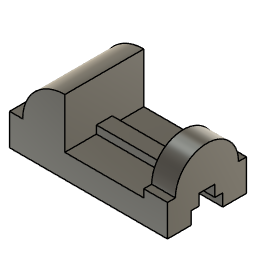
task 1 object 2 (Autodesk Fusion 360 design; units mm, degrees)
Autodesk Fusion 360 part; units mm, degrees
sketch "Sketch1" plane through (0, 0, 0) normal (0, 0, 1) x (1, 0, 0)
  line L0 (0, 0) -> (200, 0)
  line L1 (200, 0) -> (200, -100)
  line L2 (200, -100) -> (0, -100)
  line L3 (0, -100) -> (0, 0)
  dimension "d1" = 200
  dimension "d2" = 100
  constraint horizontal L0
  constraint vertical L1
  constraint horizontal L2
  constraint vertical L3
  constraint coincident L0.start L3.end
  measures "d1" distance of L0.start L0.end
  measures "d2" distance of L0.start L2.end
extrude "Extrude1" add sketch "Sketch1" along normal blind 40
sketch "Sketch2" plane through (0, 0, 40) normal (0, 0, 1) x (-1, 0, 0)
  line L0 (0, 100) -> (-200, 100)
  line L1 (-200, 100) -> (-200, 0)
  line L2 (-200, 0) -> (0, 0)
  line L3 (0, 0) -> (0, 100)
  line L4 (-200, 0) -> (-170, 0)
  line L5 (-170, 100) -> (-170, 0)
  line L6 (-200, 100) -> (-170, 100)
  constraint coincident L1.end L2.start
  constraint coincident L2 L4.end
  constraint coincident L0 L5.start
  constraint perpendicular L4 L5
  constraint coincident L0.end L1.start
extrude "Extrude2" add sketch "Sketch2" along normal blind 40 contours L0 L1 L2 L4 L5 L6
sketch "Sketch3" plane through (170, 0, 0) normal (-1, 0, 0) x (0, -1, 0)
  line L0 (0, 40) -> (100, 40)
  line L1 (100, 40) -> (100, 80)
  line L2 (100, 80) -> (0, 80)
  line L3 (0, 80) -> (0, 40)
  arc A0 (90, 40) -> (10, 40) centre (50, 40) ccw
  dimension "d7" = 80
  constraint midpoint L0 A0.centre
  constraint coincident L0 A0.end
  constraint coincident L0 A0.start
  measures "d7" diameter of A0
extrude "Extrude3" cut sketch "Sketch3" against normal blind 30 contours L0 L2 L3 A0 | L0 L1 L2 A0
sketch "Sketch4" plane through (0, 0, 0) normal (-1, 0, 0) x (0, -1, 0)
  line L0 (0, 0) -> (100, 0)
  line L1 (100, 0) -> (100, 40)
  line L2 (100, 40) -> (0, 40)
  line L3 (0, 40) -> (0, 0)
  line L4 (50, 30) -> (40, 30)
  line L5 (40, 30) -> (40, 15.5434)
  line L6 (40, 15.5434) -> (30, 15.5434)
  line L7 (30, 15.5434) -> (30, 0)
  line L8 (50, 30) -> (60, 30)
  line L9 (60, 30) -> (60, 16)
  line L10 (60, 16) -> (70, 16)
  line L11 (70, 16) -> (70, 0)
  constraint parallel L2 L4
  constraint perpendicular L4 L5
  constraint perpendicular L5 L6
  constraint perpendicular L6 L7
  constraint parallel L4 L8
  constraint perpendicular L4 L9
  constraint perpendicular L9 L10
  constraint coincident L0 L11.end
  constraint perpendicular L0 L11
extrude "Extrude4" cut sketch "Sketch4" against normal blind 200 contours L0 L4 L5 L6 L7 L8 L9 L10 L11
sketch "Sketch5" plane through (0, 0, 40) normal (0, 0, 1) x (-1, 0, 0)
  line L0 (-170, 90) -> (-170, 10)
  line L1 (-170, 10) -> (-200, 10)
  line L2 (-200, 10) -> (-200, 0)
  line L3 (-200, 0) -> (0, 0)
  line L4 (0, 0) -> (0, 100)
  line L5 (0, 100) -> (-200, 100)
  line L6 (-200, 100) -> (-200, 90)
  line L7 (-200, 90) -> (-170, 90)
  line L8 (0, 0) -> (-70, 0)
  line L9 (-70, 0) -> (-70, 100)
  line L10 (-70, 100) -> (0, 100)
  line L11 (0, 100) -> (0, 0)
  constraint horizontal L8
  constraint vertical L9
  constraint horizontal L10
  constraint vertical L11
  constraint coincident L5 L9.end
  constraint coincident L3.end L4.start
extrude "Extrude5" add sketch "Sketch5" along normal blind 55 contours L3 L4 L5 L8 L9 L10 L11
sketch "Sketch6" plane through (0, 0, 95) normal (0, 0, 1) x (-1, 0, 0)
  line L0 (0, 100) -> (-70, 100)
  line L1 (-70, 100) -> (-70, 0)
  line L2 (-70, 0) -> (0, 0)
  line L3 (0, 0) -> (0, 100)
  line L4 (0, 0) -> (-16.6169, 0)
  line L5 (-16.6169, 0) -> (-16.6169, 100)
  line L6 (-16.6169, 100) -> (0, 100)
  line L7 (0, 100) -> (0, 0)
  constraint horizontal L4
  constraint vertical L5
  constraint horizontal L6
  constraint vertical L7
  constraint coincident L0 L5.end
  constraint coincident L2.end L3.start
extrude "Extrude6" cut sketch "Sketch6" against normal blind 55 contours L0 L2 L3 L4 L5 L6 L7
sketch "Sketch7" plane through (0, -100, 0) normal (0, -1, 0) x (1, 0, 0)
  line L0 (16.6169, 40) -> (0, 40)
  line L1 (0, 40) -> (0, 0)
  line L2 (0, 0) -> (200, 0)
  line L3 (200, 0) -> (200, 40)
  line L4 (200, 40) -> (70, 40)
  line L5 (70, 40) -> (70, 95)
  line L6 (70, 95) -> (16.6169, 95)
  line L7 (16.6169, 95) -> (16.6169, 40)
  arc A0 (70, 93.3831) -> (16.6169, 40) centre (70, 40) ccw
  line L8 (70, 93.3831) -> (16.6169, 93.3831)
  constraint coincident L5 A0.start
  constraint coincident L0.start L7.end
  constraint coincident L4.end L5.start
  constraint coincident L7 L8.end
  constraint tangent A0 L8
extrude "Extrude7" cut sketch "Sketch7" against normal blind 200 contours L5 L6 L7 L8
sketch "Sketch8" plane through (0, -100, 0) normal (0, -1, 0) x (1, 0, 0)
  line L0 (70, 93.3831) -> (16.6169, 93.3831)
  line L1 (16.6169, 93.3831) -> (16.6169, 40)
  line L2 (16.6169, 40) -> (0, 40)
  line L3 (0, 40) -> (0, 0)
  line L4 (0, 0) -> (200, 0)
  line L5 (200, 0) -> (200, 40)
  line L6 (200, 40) -> (70, 40)
  line L7 (70, 40) -> (70, 93.3831)
  arc A0 (70, 93.3831) -> (16.6169, 40) centre (70, 40) ccw
  constraint coincident L7 L0.start
  constraint coincident L1.end L2.start
  constraint coincident L6.end L7.start
extrude "Extrude8" cut sketch "Sketch8" against normal blind 200 contours L0 L1 A0
sketch "Sketch9" plane through (0, 0, 40) normal (0, 0, 1) x (-1, 0, 0)
  line L0 (-70, 0) -> (-70, 100)
  line L1 (-70, 100) -> (-200, 100)
  line L2 (-200, 100) -> (-200, 90)
  line L3 (-200, 90) -> (-170, 90)
  line L4 (-170, 90) -> (-170, 10)
  line L5 (-170, 10) -> (-200, 10)
  line L6 (-200, 10) -> (-200, 0)
  line L7 (-200, 0) -> (-70, 0)
  line L8 (-170, 0) -> (-170, 40)
  line L9 (-170, 40) -> (-70, 40)
  line L10 (-170, 100) -> (-170, 60)
  line L11 (-170, 60) -> (-70, 60)
  dimension "d20" = 40
  dimension "d21" = 40
  constraint vertical L8
  constraint coincident L7 L8.start
  constraint coincident L0 L9.end
  constraint perpendicular L0 L9
  constraint coincident L1 L10.start
  constraint perpendicular L1 L10
  constraint coincident L0 L11.end
  constraint perpendicular L0 L11
  measures "d20" distance of L8.start L8.end
  measures "d21" distance of L10.start L10.end
extrude "Extrude9" cut sketch "Sketch9" against normal blind 10 contours L0 L4 L7 L8 L9 | L0 L1 L4 L10 L11
